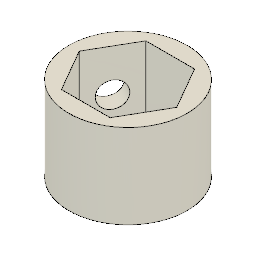
Collar v2 (Autodesk Fusion 360 design; units mm, degrees)
Autodesk Fusion 360 part; units mm, degrees
sketch "Sketch1" plane through (0, 0, 0) normal (0, 1, 0) x (1, 0, 0)
  line L0 (-2.8868, 5) -> (-5.7735, 0)
  line L1 (-5.7735, 0) -> (-2.8868, -5)
  line L2 (-2.8868, -5) -> (2.8868, -5)
  line L3 (2.8868, -5) -> (5.7735, 0)
  line L4 (5.7735, 0) -> (2.8868, 5)
  line L5 (2.8868, 5) -> (-2.8868, 5)
  circle A0 centre (0, 0) radius 7
  dimension "d1" = 5
  dimension "d2" = 14
  measures "d1" distance of A0.centre L5
  measures "d2" diameter of A0
extrude "Extrude1" add sketch "Sketch1" along normal blind 10
sketch "Sketch2" plane through (-4.3301, 0, -2.5) normal (0.866025, 0, 0.5) x (0.5, 0, -0.866025)
  line L0 (-2.8868, 0) -> (2.8868, 0)
  line L1 (2.8868, 0) -> (2.8868, 10)
  line L2 (2.8868, 10) -> (-2.8868, 10)
  line L3 (-2.8868, 10) -> (-2.8868, 0)
  circle A0 centre (0, 5) radius 1.5
  dimension "d5" = 3
  dimension "d6" = 5
  measures "d5" diameter of A0
  measures "d6" distance of origin
extrude "Extrude2" cut sketch "Sketch2" against normal through all contours A0
